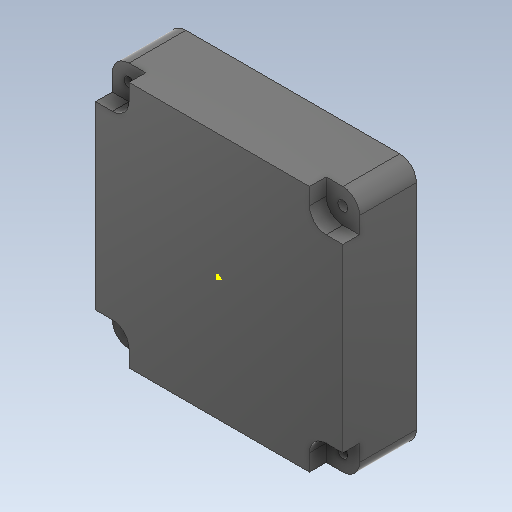
# Autodesk Inventor part: RTK-F9P-Sirius_rover
Saved by Autodesk Inventor 2020.2 (Build 242310000, 310)
## iProperties
Created: 2020-08-20
Part Number: RTK-F9P-Sirius_rover
Material: Generic
Document SubType Name: Modeling
Designer: Krishna Makhija
Density: 1 g/cm^3
Appearance: Default
Author: Krishna Makhija
Autodesk Inventor part; units mm, degrees
ref_plane "YZ Plane" through (0, 0, 0) normal (1, 0, 0) x (0, 1, 0)
ref_plane "XZ Plane" through (0, 0, 0) normal (0, 1, 0) x (-1, 0, 0)
ref_plane "XY Plane" through (0, 0, 0) normal (0, 0, 1) x (1, 0, 0)
sketch "Sketch1" plane through (0, 0, 0) normal (0, 0, 1) x (1, 0, 0)
  line L0 (37.0001, -37.0002) -> (-37.0001, -37.0002)
  line L1 (-37.0001, -37.0002) -> (-37.0001, 37.0002)
  line L2 (-37.0001, 37.0002) -> (37.0001, 37.0002)
  line L3 (37.0001, 37.0002) -> (37.0001, -37.0002)
  line L4 (69.0001, -5.0002) -> (-5.0001, 69.0002) construction
  circle A0 centre (32, 32) radius 1.5
  circle A1 centre (32, -32) radius 1.5
  circle A2 centre (-32, 32) radius 1.5
  line L5 (5.0001, -69.0002) -> (-69.0001, 5.0002) construction
  circle A3 centre (-32, -32) radius 1.5
  line L6 (37.0001, -101.0002) -> (-37.0001, -26.9998) construction
  line L7 (5.0001, -69.0002) -> (-69.0001, 5.0002) construction
  constraints: 16 end point, 4 centre point, 2 parallel, 1 horizontal, 1 perpendicular
extrude "Extrusion1" add sketch "Sketch1" along normal blind 22
fillet "Fillet1" radius 5 4 edges at (-37.0001, 37.0002, 11) (37.0001, 37.0002, 11) (37.0001, -37.0002, 11) (-37.0001, -37.0002, 11)
sketch "Sketch2" plane through (0, 0, 0) normal (0, 0, -1) x (-1, 0, 0)
  point P0 (0, 0)
sketch "Sketch4" plane through (0, 0, 22) normal (0, 0, 1) x (1, 0, 0)
  point P0 (0, 0)
sketch "Sketch5" plane through (0, 0, 22) normal (0, 0, 1) x (1, 0, 0)
  line L0 (-37.0001, 32.0002) -> (-37.0001, -32.0002) projected
  line L1 (-26.9999, 37.0018) -> (-37.0001, 37.0018)
  line L2 (-37.0001, 37.0018) -> (-37.0001, 26.9982)
  line L3 (-37.0001, 26.9982) -> (-26.9999, 26.9982)
  line L4 (-26.9999, 26.9982) -> (-26.9999, 37.0018)
  circle A0 centre (-32, 32) radius 1.5 projected
  line L5 (-26.9999, 37.0018) -> (-37.0001, 26.9982) construction
  line L6 (-37.0001, 37.0018) -> (-26.9999, 26.9982) construction
  line L7 (37.0001, 37.0018) -> (26.9999, 37.0018)
  line L8 (26.9999, 37.0018) -> (26.9999, 26.9982)
  line L9 (26.9999, 26.9982) -> (37.0001, 26.9982)
  line L10 (37.0001, 26.9982) -> (37.0001, 37.0018)
  line L11 (37.0001, 37.0018) -> (26.9999, 26.9982) construction
  line L12 (26.9999, 37.0018) -> (37.0001, 26.9982) construction
  line L13 (-26.9999, -26.9982) -> (-37.0001, -26.9982)
  line L14 (-37.0001, -26.9982) -> (-37.0001, -37.0018)
  line L15 (-37.0001, -37.0018) -> (-26.9999, -37.0018)
  line L16 (-26.9999, -37.0018) -> (-26.9999, -26.9982)
  line L17 (-26.9999, -26.9982) -> (-37.0001, -37.0018) construction
  line L18 (-37.0001, -26.9982) -> (-26.9999, -37.0018) construction
  line L19 (37.0001, -26.9982) -> (26.9999, -37.0018) construction
  line L20 (37.0001, -37.0018) -> (37.0001, -26.9982)
  line L21 (26.9999, -37.0018) -> (37.0001, -37.0018)
  line L22 (26.9999, -26.9982) -> (26.9999, -37.0018)
  line L23 (37.0001, -26.9982) -> (26.9999, -26.9982)
  line L24 (26.9999, -26.9982) -> (37.0001, -37.0018) construction
  point P0 (0, 0)
  constraints: 48 end point, 8 parallel, 4 horizontal, 4 perpendicular, 2 midpoint, 1 point on line
extrude "Extrusion2" cut sketch "Sketch5" against normal blind 5 contours L2 L1 L4 L3 L0 | L13 L16 L15 L14 L0 | A0 | L10 L9 L8 L7 | L21 L22 L23 L20
fillet "Fillet2" radius 5 4 edges at (-26.9999, 26.9982, 19.5) (26.9999, 26.9982, 19.5) (-26.9999, -26.9982, 19.5) (26.9999, -26.9982, 19.5)
sketch "Sketch6" plane through (0, 0, 22) normal (0, 0, 1) x (1, 0, 0)
  line L0 (96.2626, 67.9332) -> (202.4541, 67.9332) construction
  line L1 (202.4541, 67.9332) -> (202.4541, -70.892) construction
  line L2 (202.4541, -70.892) -> (96.2626, -70.892) construction
  line L3 (96.2626, -70.892) -> (96.2626, 67.9332) construction
  point P0 (0, 0)
  constraints: 2 other
decal "Decal3"
body "Solid1"
